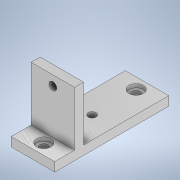
# Autodesk Inventor part: UEOM L mount Vertical
Saved by Autodesk Inventor 2020 (Build 240168000, 168)
## iProperties
Created: 2020-10-29
Part Number: UEOM L mount Vertical
Material: Generic
Document SubType Name: Modeling
Designer: Austin
Density: 1 g/cm^3
Appearance: Machined - Aluminum
Author: Austin
Autodesk Inventor part; units mm, degrees
ref_plane "YZ Plane" through (0, 0, 0) normal (1, 0, 0) x (0, 1, 0)
ref_plane "XZ Plane" through (0, 0, 0) normal (0, 1, 0) x (-1, 0, 0)
ref_plane "XY Plane" through (0, 0, 0) normal (0, 0, 1) x (1, 0, 0)
sketch "Sketch14" plane through (0, 0, 0) normal (0, 1, 0) x (-1, 0, 0)
  line L0 (12, 14) -> (-12, 14)
  line L1 (-12, 14) -> (-12, -14)
  line L2 (-12, -14) -> (12, -14)
  line L3 (12, -14) -> (12, 14)
  line L4 (12, 14) -> (-12, -14) construction
  line L5 (-12, 14) -> (12, -14) construction
  line L6 (12, 14) -> (-12, 14)
  line L7 (-12, 14) -> (-12, 30)
  line L8 (-12, 30) -> (12, 30)
  line L9 (12, 30) -> (12, 14)
  line L10 (-12, -14) -> (12, -14)
  line L11 (12, -14) -> (12, -33)
  line L12 (12, -33) -> (-12, -33)
  line L13 (-12, -33) -> (-12, -14)
  point P0 (0, 0)
  point P1 (12, -14)
  dimension "d93" = 28
  dimension "d94" = 24
  dimension "d95" = 16
  dimension "d111" = 19
  constraints: 28 end point, 6 parallel, 3 horizontal, 3 perpendicular, 2 midpoint
  measures "d93" distance of L2.end L0.start
  measures "d94" distance of L0.start L0.end
  measures "d95" distance between parallel lines of L0 L8
  measures "d111" distance of L12.end L1.end
extrude "Extrusion8" add sketch "Sketch14" along normal blind 5
sketch "Sketch17" plane through (0, 5, 0) normal (0, 1, 0) x (1, 0, 0)
  line L0 (-12, -30) -> (12, -30) projected
  line L1 (12, 33) -> (-12, 33) projected
  point P0 (0, 0)
  point P1 (0, 27)
  point P2 (0, -24)
  dimension "d119" = 0
  dimension "d121" = 6
  dimension "d122" = 0
  dimension "d125" = 6
  measures "d119" horizontal distance of point (0, 0) point (0, 27)
  measures "d121" distance from line of L0 point (0, -24)
  measures "d122" horizontal distance of point (0, 0) point (0, -24)
  measures "d125" distance from line of L1 point (0, 27)
hole "Hole8" at (0, 5, -27) at (0, 5, 24) direction (0, -1, 0) diameter 4.305 end through all counterbore diameter 7.938 counterbore depth 2 clearance for "Socket Head Cap Screw" size "#8" standard "Ansi Unified Screw Threads"
sketch "Sketch18" plane through (0, 5, 0) normal (0, 1, 0) x (1, 0, 0)
  line L0 (12, -30) -> (12, 33) projected
  line L1 (-12, 33) -> (-12, -30) projected
  line L2 (12, -14) -> (-12, -14)
  line L3 (-12, -14) -> (-12, -19)
  line L4 (-12, -19) -> (12, -19)
  line L5 (12, -19) -> (12, -14)
  point P0 (0, 0)
  point P1 (-12, -14)
  dimension "d126" = 5
  dimension "d127" = 14
  constraints: 8 end point, 2 parallel, 2 point on line, 1 horizontal, 1 perpendicular
  measures "d126" distance between parallel lines of L4 L2
  measures "d127" distance from line of L2 point (0, 0)
extrude "Extrusion10" add sketch "Sketch18" along normal blind 30
sketch "Sketch19" plane through (-12, 5, 19) normal (0, 0, 1) x (1, 0, 0)
  line L0 (0, 0) -> (24, 0) projected
  line L1 (0, 0) -> (0, 30) projected
  point P0 (12, -5)
  point P1 (12, 24.659)
  dimension "d138" = 24.659
  dimension "d148" = 12
  measures "d138" distance from line of L0 point (12, 24.659)
  measures "d148" distance from line of L1 point (12, 24.659)
hole "Hole9" at (0, 29.659, 19) direction (0, 0, -1) diameter 4.3 depth 11.8 clearance for "Socket Head Cap Screw" size "M4" standard "Ansi Metric M Profile"
sketch "Sketch20" plane through (0, 0, 0) normal (0, -1, 0) x (1, 0, 0)
  line L0 (-12, 14) -> (12, 14) projected
  point P0 (0, 0)
  point P1 (0, -2.678)
  dimension "d146" = 16.678
  dimension "d147" = 0
  measures "d146" distance from line of L0 point (0, -2.678)
  measures "d147" horizontal distance of point (0, 0) point (0, -2.678)
hole "Hole10" at (0, 0, -2.678) direction (0, 1, 0) diameter 4.3 depth 11.8 counterbore diameter 8 counterbore depth 2 clearance for "Socket Head Cap Screw" size "M4" standard "Ansi Metric M Profile"
equation "\"d138\" = a"
equation "\"d146\" = b"
equation "\"LASER_HOLE_HEIGHT\" = 16.7"
equation "\"a\" = 24.659"
equation "\"b\" = 16.678"
body "Solid2"
